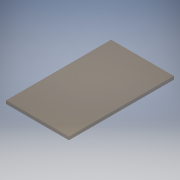
# Autodesk Inventor part: MotorMountDCB
Saved by Autodesk Inventor 2019 (Build 230136000, 136)
## iProperties
Created: 2019-01-19
Part Number: MotorMountDCB
Material: Polycarbonate, Smoke
Document SubType Name: Modeling
Designer: nxgam
Density: 1.2 g/cm^3
Appearance: Polycarbonate - Smoked
Author: nxgam
Autodesk Inventor part; units mm, degrees
ref_plane "YZ Plane" through (0, 0, 0) normal (1, 0, 0) x (0, 1, 0)
ref_plane "XZ Plane" through (0, 0, 0) normal (0, 1, 0) x (-1, 0, 0)
ref_plane "XY Plane" through (0, 0, 0) normal (0, 0, 1) x (1, 0, 0)
sketch "Sketch1" plane through (0, 0, 0) normal (0, 1, 0) x (-1, 0, 0)
  line L0 (-27.3558, 45.72) -> (27.3558, 45.72)
  line L1 (27.3558, 45.72) -> (27.3558, -45.72)
  line L2 (27.3558, -45.72) -> (-27.3558, -45.72)
  line L3 (-27.3558, -45.72) -> (-27.3558, 45.72)
  line L4 (-27.3558, 45.72) -> (27.3558, -45.72) construction
  line L5 (27.3558, 45.72) -> (-27.3558, -45.72) construction
  point P0 (0, 0)
  dimension "d0" = 54.7116
  dimension "d1" = 91.44
  constraints: 12 end point, 2 midpoint, 2 parallel, 1 horizontal, 1 perpendicular
  measures "d0" distance of L1.end L2.end
  measures "d1" distance of L0.end L1.end
extrude "Extrusion1" add sketch "Sketch1" along normal blind 2.794
sketch "Sketch2" plane through (0, 2.794, 0) normal (0, 1, 0) x (1, 0, 0)
  circle A0 centre (-6.3442, 0) radius 6 construction
  circle A1 centre (0.6558, 0) radius 18.4 construction
  circle A2 centre (-7.0942, -13.4234) radius 1.25 construction
  circle A3 centre (-12.7676, -7.75) radius 1.25 construction
  circle A4 centre (-12.7676, 7.75) radius 1.25 construction
  circle A5 centre (-7.0942, 13.4234) radius 1.25 construction
  circle A6 centre (0.6558, 15.5) radius 1.25 construction
  circle A7 centre (14.0792, 7.75) radius 1.25 construction
  circle A8 centre (16.1558, 0) radius 1.25 construction
  circle A9 centre (14.0792, -7.75) radius 1.25 construction
  circle A10 centre (0.6558, -15.5) radius 1.25 construction
  spline S0 degree 3 poles (-6.3442, -8.58) (-7.0027, -8.6329) (-7.0027, -9.0013) (-6.3442, -9.6852) knots -1 -1 -1 -1 0 0 0 0 construction
  arc A11 (-6.3442, -9.6852) -> (-6.3442, 9.6852) centre (0.6558, 0) ccw construction
  spline S1 degree 3 poles (-6.3442, 9.6852) (-7.0027, 9.0013) (-7.0027, 8.6329) (-6.3442, 8.58) knots -1 -1 -1 -1 0 0 0 0 construction
  arc A12 (-6.3442, -8.58) -> (-6.3442, 8.58) centre (-6.3442, 0) ccw construction
  circle A13 centre (-6.3442, 0) radius 6.223
  point P0 (0, 0)
  dimension "d4" = 12.446
  constraints: 14 centre point, 7 coincident, 4 point on circle, 2 vertical alignment, 34 other
  measures "d4" diameter of A13
hole "Hole1" at (0.6558, 2.794, -15.5) at (0.6558, 2.794, 15.5) at (14.0792, 2.794, -7.75) at (14.0792, 2.794, 7.75) at (-12.7676, 2.794, -7.75) at (-12.7676, 2.794, 7.75) direction (0, -1, 0) diameter 3 end through all
extrude "Extrusion2" cut sketch "Sketch2" against normal blind 25.4
sketch "Sketch3" plane through (0, 2.794, 0) normal (0, 1, 0) x (1, 0, 0)
  point P0 (0, 0)
sketch "Sketch4" plane through (0, 0, 0) normal (0, -1, 0) x (1, 0, 0)
  arc A0 (8.0816, -16.5469) -> (10.5912, -15.0645) centre (9.1558, -15.5) ccw
  arc A1 (10.5912, -15.0645) -> (10.5912, 15.0645) centre (0, 0) ccw
  arc A2 (10.5912, 15.0645) -> (8.0816, 16.5469) centre (9.1558, 15.5) ccw
  arc A3 (8.0816, 16.5469) -> (8.0816, -16.5469) centre (0, 0) ccw
  circle A4 centre (-21.8442, -15.5) radius 1.5
  circle A5 centre (-21.8442, 15.5) radius 1.5
  arc A6 (-27.3558, -42.545) -> (-24.1808, -45.72) centre (-24.1808, -42.545) ccw
  line L0 (-27.3558, -42.545) -> (-27.3558, 42.545)
  arc A7 (-24.1808, 45.72) -> (-27.3558, 42.545) centre (-24.1808, 42.545) ccw
  line L1 (-24.1808, 45.72) -> (24.1808, 45.72)
  arc A8 (27.3558, 42.545) -> (24.1808, 45.72) centre (24.1808, 42.545) ccw
  line L2 (27.3558, 42.545) -> (27.3558, -42.545)
  arc A9 (24.1808, -45.72) -> (27.3558, -42.545) centre (24.1808, -42.545) ccw
  line L3 (24.1808, -45.72) -> (-24.1808, -45.72)
  circle A10 centre (9.1558, -15.5) radius 3.25
  circle A11 centre (9.1558, 15.5) radius 3.25
  point P0 (0, 0)
  dimension "d14" = 6.5
  dimension "d15" = 6.5
  constraints: 16 point on circle, 12 centre point, 8 end point, 2 coincident, 2 horizontal, 2 vertical, 32 other
  measures "d14" diameter of A11
  measures "d15" diameter of A10
extrude "Extrusion3" cut sketch "Sketch4" against normal blind 25.4 contours A3 A10 A1 A0 | A0 A1 A10 A3 | A11 A1 A2 A3 | A3 A2 A1 A11 | A4 | A5
fillet "Fillet1" radius 3.175 4 edges at (-27.3558, 1.397, -45.72) (-27.3558, 1.397, 45.72) (27.3558, 1.397, 45.72) (27.3558, 1.397, -45.72)
equation "\"d15\" = d14"
body "Solid1"
